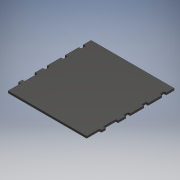
# Autodesk Inventor part: BA09
Saved by Autodesk Inventor 2017 (Build 210142000, 142)
## iProperties
Created: 2019-05-29
Part Number: BA09
Material: Wood (Cherry)
Document SubType Name: Modeling
Designer: Dell
Density: 0.63 g/cm^3
Appearance: Smooth - Black
Author: Dell
Autodesk Inventor part; units mm, degrees
ref_plane "YZ Plane" through (0, 0, 0) normal (1, 0, 0) x (0, 1, 0)
ref_plane "XZ Plane" through (0, 0, 0) normal (0, 1, 0) x (-1, 0, 0)
ref_plane "XY Plane" through (0, 0, 0) normal (0, 0, 1) x (1, 0, 0)
sketch "Sketch1" plane through (0, 0, 0) normal (0, 0, 1) x (1, 0, 0)
  line L0 (0, 0) -> (525.78, 0)
  line L1 (525.78, 0) -> (525.78, 355.6)
  line L2 (525.78, 355.6) -> (0, 355.6)
  line L3 (0, 355.6) -> (0, 0)
  dimension "d0" = 525.78
  dimension "d1" = 355.6
  constraints: 8 end point, 2 parallel, 1 horizontal, 1 perpendicular
  measures "d0" distance of L2.end L1.end
  measures "d1" distance of L2.end L0.start
extrude "Extrusion1" add sketch "Sketch1" along normal blind 12.7
sketch "Sketch2" plane through (0, 0, 12.7) normal (0, 0, 1) x (1, 0, 0)
  line L0 (525.78, 0) -> (525.78, 355.6) projected
  line L1 (525.78, 306.07) -> (511.81, 306.07)
  line L2 (511.81, 306.07) -> (511.81, 278.13)
  line L3 (511.81, 278.13) -> (525.78, 278.13)
  line L4 (525.78, 278.13) -> (525.78, 306.07)
  line L5 (525.78, 191.135) -> (511.81, 191.135)
  line L6 (511.81, 191.135) -> (511.81, 164.465)
  line L7 (511.81, 164.465) -> (525.78, 164.465)
  line L8 (525.78, 164.465) -> (525.78, 191.135)
  line L9 (525.78, 77.47) -> (511.81, 77.47)
  line L10 (511.81, 77.47) -> (511.81, 49.53)
  line L11 (511.81, 49.53) -> (525.78, 49.53)
  line L12 (525.78, 49.53) -> (525.78, 77.47)
  line L13 (0, 306.07) -> (13.97, 306.07)
  line L14 (13.97, 306.07) -> (13.97, 278.13)
  line L15 (13.97, 278.13) -> (0, 278.13)
  line L16 (0, 278.13) -> (0, 306.07)
  line L17 (0, 355.6) -> (0, 0) projected
  line L18 (0, 164.465) -> (13.97, 164.465)
  line L19 (13.97, 164.465) -> (13.97, 191.135)
  line L20 (13.97, 191.135) -> (0, 191.135)
  line L21 (0, 191.135) -> (0, 164.465)
  line L22 (0, 77.47) -> (13.97, 77.47)
  line L23 (13.97, 77.47) -> (13.97, 49.53)
  line L24 (13.97, 49.53) -> (0, 49.53)
  line L25 (0, 49.53) -> (0, 77.47)
  point P0 (0, 177.8)
  point P1 (525.78, 177.8)
  dimension "d4" = 13.97
  dimension "d5" = 13.97
  dimension "d6" = 27.94
  dimension "d7" = 26.67
  dimension "d8" = 27.94
  dimension "d9" = 49.53
  dimension "d10" = 49.53
  constraints: 48 end point, 12 parallel, 8 point on line, 6 horizontal, 6 perpendicular, 5 horizontal alignment, 4 midpoint, 4 vertical alignment
  measures "d4" distance of L13.start L13.end
  measures "d5" distance of L1.start L1.end
  measures "d6" distance of L13.end L14.end
  measures "d7" distance of L18.end L19.end
  measures "d8" distance of L22.end L23.end
  measures "d9" distance of L17.start L13.start
  measures "d10" distance of L17.end L24.end
extrude "Extrusion2" cut sketch "Sketch2" against normal through all
sketch "Sketch3" plane through (0, 0, 12.7) normal (0, 0, 1) x (1, 0, 0)
  line L0 (0, 0) -> (525.78, 0)
  line L1 (525.78, 0) -> (525.78, -184.15)
  line L2 (525.78, -184.15) -> (0, -184.15)
  line L3 (0, -184.15) -> (0, 0)
  line L4 (525.78, 355.6) -> (0, 355.6) projected
  line L5 (0, -78.105) -> (13.97, -78.105)
  line L6 (13.97, -78.105) -> (13.97, -106.045)
  line L7 (13.97, -106.045) -> (0, -106.045)
  line L8 (0, -106.045) -> (0, -78.105)
  line L9 (525.78, -78.105) -> (511.81, -78.105)
  line L10 (511.81, -78.105) -> (511.81, -106.045)
  line L11 (511.81, -106.045) -> (525.78, -106.045)
  line L12 (525.78, -106.045) -> (525.78, -78.105)
  line L13 (525.78, -79.375) -> (539.75, -79.375)
  line L14 (539.75, -79.375) -> (539.75, -104.775)
  line L15 (539.75, -104.775) -> (525.78, -104.775)
  line L16 (525.78, -104.775) -> (525.78, -79.375)
  line L17 (0, -79.375) -> (-13.97, -79.375)
  line L18 (-13.97, -79.375) -> (-13.97, -104.775)
  line L19 (-13.97, -104.775) -> (0, -104.775)
  line L20 (0, -104.775) -> (0, -79.375)
  point P0 (13.97, 49.53)
  point P1 (511.81, 49.53)
  point P2 (525.78, -92.075)
  point P3 (0, -92.075)
  dimension "d13" = 539.75
  dimension "d16" = 27.94
  dimension "d17" = 27.94
  dimension "d18" = 25.4
  dimension "d19" = 13.97
  dimension "d20" = 13.97
  dimension "d21" = 25.4
  constraints: 40 end point, 10 parallel, 6 midpoint, 5 horizontal, 5 perpendicular, 4 point on line, 2 vertical alignment, 1 coincident
  measures "d13" distance between parallel lines of L4 L2
  measures "d16" distance of L5.end L6.end
  measures "d17" distance of L9.end L10.end
  measures "d18" distance of L13.end L14.end
  measures "d19" distance of L13.start L13.end
  measures "d20" distance of L19.end L18.end
  measures "d21" distance of L18.end L17.end
extrude "Extrusion3" add sketch "Sketch3" against normal blind 12.7
sketch "Sketch4" plane through (0, 0, 12.7) normal (0, 0, 1) x (1, 0, 0)
  line L0 (525.78, 49.53) -> (525.78, -79.375) projected
  line L1 (525.78, -184.15) -> (0, -184.15) projected
  line L2 (525.78, 0) -> (511.81, 0)
  line L3 (511.81, 0) -> (511.81, -184.15)
  line L4 (511.81, -184.15) -> (525.78, -184.15)
  line L5 (525.78, -184.15) -> (525.78, 0)
  line L6 (525.78, -79.375) -> (539.75, -79.375) projected
  line L7 (525.78, -79.375) -> (511.81, -79.375)
  line L8 (511.81, -79.375) -> (511.81, -104.775)
  line L9 (511.81, -104.775) -> (525.78, -104.775)
  line L10 (525.78, -104.775) -> (525.78, -79.375)
  line L11 (0, 0) -> (13.97, 0)
  line L12 (13.97, 0) -> (13.97, -184.15)
  line L13 (13.97, -184.15) -> (0, -184.15)
  line L14 (0, -184.15) -> (0, 0)
  line L15 (0, -79.375) -> (13.97, -79.375)
  line L16 (13.97, -79.375) -> (13.97, -104.775)
  line L17 (13.97, -104.775) -> (0, -104.775)
  line L18 (0, -104.775) -> (0, -79.375)
  line L19 (525.78, -79.375) -> (539.75, -79.375)
  line L20 (539.75, -79.375) -> (539.75, -104.775)
  line L21 (539.75, -104.775) -> (525.78, -104.775)
  line L22 (525.78, -104.775) -> (525.78, -79.375)
  line L23 (0, -104.775) -> (-13.97, -104.775) projected
  line L24 (0, -104.775) -> (-13.97, -104.775)
  line L25 (-13.97, -104.775) -> (-13.97, -79.375)
  line L26 (-13.97, -79.375) -> (0, -79.375)
  line L27 (0, -79.375) -> (0, -104.775)
  line L28 (-13.97, -79.375) -> (-13.97, -104.775) projected
  point P0 (0, -104.775)
  point P1 (511.81, 49.53)
  point P2 (13.97, 49.53)
  constraints: 48 end point, 12 parallel, 8 point on line, 6 horizontal, 6 perpendicular, 2 coincident, 2 vertical alignment, 1 horizontal alignment
extrude "Extrusion4" cut sketch "Sketch4" against normal through all contours L0 L7 L3 L2 | L6 L20 L21 L5 | L5 L1 L3 L9 | L1 L14 L17 L12 | L23 L25 L26 L14 | L15 L14 L11 L12
body "Solid1"
